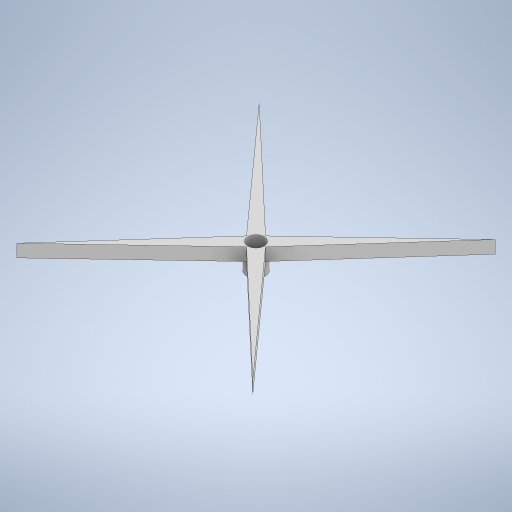
# Autodesk Inventor part: Ventilador Pieza extra de ensamble SEBASTIAN BERMUDEZ
Saved by Autodesk Inventor 2024.2 (Build 282272000, 272)
## iProperties
Created: 2024-03-31
Part Number: Ventilador Pieza extra de ensamble SEBASTIAN BERMUDEZ
Material: Generic
Document SubType Name: Modeling
Designer: sberl
Density: 1 g/cm^3
Appearance: Default
Author: sberl
Autodesk Inventor part; units mm, degrees
ref_plane "YZ Plane" through (0, 0, 0) normal (1, 0, 0) x (0, 1, 0)
ref_plane "XZ Plane" through (0, 0, 0) normal (0, 1, 0) x (-1, 0, 0)
ref_plane "XY Plane" through (0, 0, 0) normal (0, 0, 1) x (1, 0, 0)
sketch "Sketch1" plane through (0, 0, 0) normal (0, 1, 0) x (-1, 0, 0)
  circle A0 centre (0, 0) radius 6.5
  circle A1 centre (0, 0) radius 7.5
  dimension "d0" = 13
  dimension "d1" = 15
  constraints: 2 centre point, 2 coincident
  measures "d0" diameter of A0
  measures "d1" diameter of A1
extrude "Extrusion1" add sketch "Sketch1" along normal blind 10
sketch "Sketch2" plane through (0, 10, 0) normal (0, 1, 0) x (1, 0, 0)
  line L0 (-93.2796, -95.8103) -> (93.2796, 95.8103) construction
  line L1 (93.2796, -95.8103) -> (-93.2796, 95.8103) construction
  circle A0 centre (0, 0) radius 7.5 projected
  line L2 (-7.5, 0) -> (-93.2796, 95.8103)
  line L3 (-93.2796, 95.8103) -> (0, 7.5)
  line L4 (0, 7.5) -> (93.2796, 95.8103)
  line L5 (93.2796, 95.8103) -> (7.5, 0)
  line L6 (7.5, 0) -> (93.2796, -95.8103)
  line L7 (93.2796, -95.8103) -> (0, -7.5)
  line L8 (0, -7.5) -> (-93.2796, -95.8103)
  line L9 (-93.2796, -95.8103) -> (-7.5, 0)
  constraints: 20 end point, 4 parallel, 4 point on circle, 2 midpoint
extrude "Extrusion2" add sketch "Sketch2" along normal blind 10
sketch "Sketch3" plane through (0, 10, 0) normal (0, -1, 0) x (1, 0, 0)
  point P0 (0, 0)
sketch "Sketch4" plane through (0, 20, 0) normal (0, 1, 0) x (1, 0, 0)
  circle A0 centre (0, 0) radius 6.5
  constraints: 1 centre point, 1 coincident
extrude "Extrusion3" cut sketch "Sketch4" against normal through all
body "Solid1"
